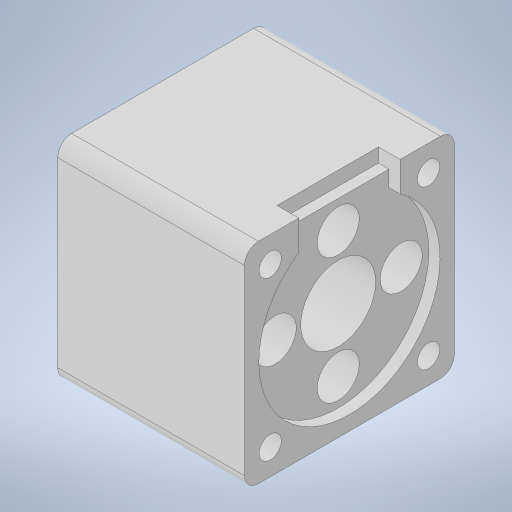
# Autodesk Inventor part: NewPart1_ver6
Saved by Autodesk Inventor 2024 (Build 280153000, 153)
## iProperties
Created: 2025-06-25
Part Number: NewPart1_ver6
Material: 一般
Document SubType Name: Modeling
Designer: HosodaLab2
Density: 1 g/cm^3
Appearance: 既定
Author: HosodaLab2
Autodesk Inventor part; units mm, degrees
ref_plane "YZ Plane" through (0, 0, 0) normal (1, 0, 0) x (0, 1, 0)
ref_plane "XZ Plane" through (0, 0, 0) normal (0, 1, 0) x (-1, 0, 0)
ref_plane "XY Plane" through (0, 0, 0) normal (0, 0, 1) x (1, 0, 0)
sketch "スケッチ4" plane through (0, 0, 0) normal (0, 1, 0) x (-1, 0, 0)
  line L0 (0, 0) -> (-30, 0)
  line L1 (-30, 0) -> (-30, -30)
  line L2 (-30, -30) -> (0, -30)
  line L3 (0, -30) -> (0, 0)
  dimension "d6" = 30
  dimension "d7" = 30
  constraints: 8 end point, 2 parallel, 1 horizontal, 1 perpendicular
  measures "d6" distance of L2.end L1.end
  measures "d7" distance of L1.end L0.end
extrude "押し出し2" add sketch "スケッチ4" along normal blind 26.7
sketch "スケッチ5" plane through (0, 26.7, 0) normal (0, 1, 0) x (1, 0, 0)
  circle A0 centre (15, 15) radius 12.95
  line L0 (0, 30) -> (0, 0) projected
  line L1 (30, 30) -> (0, 30) projected
  line L2 (7.75, 4.2697) -> (22.25, 4.2697)
  line L3 (22.25, 4.2697) -> (22.25, -0.093)
  line L4 (22.25, -0.093) -> (7.75, -0.093)
  line L5 (7.75, -0.093) -> (7.75, 4.2697)
  point P0 (0, 15)
  point P1 (15, 30)
  point P2 (7.75, 2.0883)
  point P3 (22.25, 4.2697)
  dimension "d10" = 25.9
  dimension "d28" = 14.5
  dimension "d29" = 7.25
  constraints: 8 end point, 3 midpoint, 2 parallel, 1 horizontal, 1 horizontal alignment, 1 perpendicular, 1 vertical alignment, 3 other
  measures "d28" distance from line of L3 point (7.75, 2.088)
  measures "d29" distance from line of L3 point (15, 15)
sketch "スケッチ6" plane through (0, 26.7, 0) normal (0, 1, 0) x (1, 0, 0)
  circle A0 centre (15, 15) radius 12.95 projected
  line L0 (30, 0) -> (30, 30) construction
  line L1 (30, 30) -> (0, 30) construction
  line L2 (0, 0) -> (30, 0) construction
  circle A1 centre (24.5802, 2.4198) radius 0 construction
  circle A2 centre (15, 15) radius 16 construction
  line L3 (30, 0) -> (0, 30) construction
  line L4 (0, 30) -> (0, 0) construction
  line L5 (0, 0) -> (30, 30) construction
  point P0 (24.5802, 2.4198)
  point P1 (3.6863, 3.6863)
  point P2 (3.6863, 26.3137)
  point P3 (26.3137, 26.3137)
  point P4 (26.3137, 3.6863)
  dimension "d61" = 32
  constraints: 4 end point, 4 point on circle, 4 point on line, 2 coincident, 1 centre point, 2 other
  measures "d61" diameter of A2
fillet "フィレット1" radius 2 4 edges at (0, 13.35, -30) (0, 13.35, 0) (30, 13.35, 0) (30, 13.35, -30)
extrude "押し出し3" cut sketch "スケッチ5" against normal blind 1.6
sketch "スケッチ7" plane through (0, 0, 0) normal (0, -1, 0) x (1, 0, 0)
  line L0 (0, -28) -> (0, -2) projected
  line L1 (28, -30) -> (2, -30) projected
  point P0 (0, 0)
  point P1 (15, -15)
  point P2 (0, -15)
  point P3 (15, -30)
  constraints: 2 midpoint, 1 horizontal alignment, 1 vertical alignment
hole "穴3" at (15, 0, -15) direction (0, 1, 0) diameter 10.7 end through all
sketch "スケッチ8" plane through (0, 0, 0) normal (0, -1, 0) x (1, 0, 0)
  line L0 (0, -28) -> (0, -2) projected
  line L1 (28, -30) -> (2, -30) projected
  circle A0 centre (15, -15) radius 9
  point P0 (0, 0)
  point P1 (0, -15)
  point P2 (15, -30)
  point P3 (15, -24)
  point P4 (6, -15)
  point P5 (15, -6)
  point P6 (24, -15)
  dimension "d39" = 18
  constraints: 4 point on circle, 2 midpoint, 1 centre point, 1 coincident, 1 horizontal alignment, 1 vertical alignment
  measures "d39" diameter of A0
hole "穴4" at (15, 0, -15) at (15, 0, -24) at (6, 0, -15) at (15, 0, -6) at (24, 0, -15) direction (0, 1, 0) diameter 3.2 end through all
sketch "スケッチ9" plane through (0, 25.1, 0) normal (0, 1, 0) x (1, 0, 0)
  circle A0 centre (15, 6) radius 1.6 projected
  circle A1 centre (6, 15) radius 1.6 projected
  circle A2 centre (15, 24) radius 1.6 projected
  circle A3 centre (24, 15) radius 1.6 projected
  point P0 (0, 0)
  constraints: 4 coincident
hole "穴5" at (15, 25.1, -6) at (6, 25.1, -15) at (15, 25.1, -24) at (24, 25.1, -15) direction (0, -1, 0) diameter 6 depth 15 tip angle 118
sketch "スケッチ10" plane through (0, 26.7, 0) normal (0, 1, 0) x (1, 0, 0)
  circle A0 centre (24.5802, 2.4198) radius 1.1 projected
  circle A1 centre (2.4198, 2.4198) radius 1.1 projected
  circle A2 centre (2.4198, 24.5802) radius 1.1 projected
  circle A3 centre (24.5802, 24.5802) radius 1.1 projected
  point P0 (0, 0)
  constraints: 4 coincident
hole "穴6" [suppressed]
hole "穴7" at (3.6863, 26.7, -3.6863) at (3.6863, 26.7, -26.3137) at (26.3137, 26.7, -26.3137) at (26.3137, 26.7, -3.6863) direction (0, -1, 0) diameter 3.2 end through all
sketch "スケッチ11" plane through (0, 25.1, 0) normal (0, 1, 0) x (1, 0, 0)
  line L0 (7.75, 0) -> (7.75, 4.2697) projected
  line L1 (22.25, 0) -> (7.75, 0)
  line L2 (7.75, 0) -> (7.75, 2)
  line L3 (7.75, 2) -> (22.25, 2)
  line L4 (22.25, 2) -> (22.25, 0)
  dimension "d72" = 2
  constraints: 8 end point, 2 parallel, 1 horizontal, 1 perpendicular, 1 point on line
  measures "d72" distance between parallel lines of L3 L1
extrude "押し出し5" cut sketch "スケッチ11" against normal blind 1.5
